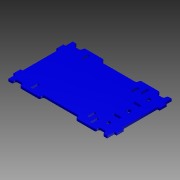
# Autodesk Inventor part: OpenROV 2.3 Dev EChassis Main Plate
Saved by Autodesk Inventor 2012 (Build 160160000, 160)
## iProperties
Created: 2011-12-20
Part Number: OpenROV 2.3 Dev EChassis Main Plate
Document SubType Name: Modeling
Designer: user
Density: 1 g/cm^3
Material: Default
Author: user
Autodesk Inventor part; units mm, degrees
ref_plane "YZ Plane" through (0, 0, 0) normal (1, 0, 0) x (0, 1, 0)
ref_plane "XZ Plane" through (0, 0, 0) normal (0, 1, 0) x (-1, 0, 0)
ref_plane "XY Plane" through (0, 0, 0) normal (0, 0, 1) x (1, 0, 0)
sketch "Sketch1" plane through (0, 0, 0) normal (0, 0, 1) x (1, 0, 0)
  line L0 (138, 80) -> (141, 80)
  line L1 (141, 80) -> (141, 70)
  line L2 (141, 70) -> (138, 70)
  line L3 (138, 10) -> (141, 10)
  line L4 (141, 10) -> (141, 20)
  line L5 (141, 20) -> (138, 20)
  line L6 (138, 80) -> (138, 90)
  line L7 (138, 20) -> (138, 70)
  line L8 (0, 80) -> (-3, 80)
  line L9 (-3, 80) -> (-3, 70)
  line L10 (-3, 70) -> (0, 70)
  line L11 (0, 20) -> (-3, 20)
  line L12 (-3, 20) -> (-3, 10)
  line L13 (-3, 10) -> (0, 10)
  line L14 (0, 90) -> (0, 80)
  line L15 (0, 70) -> (0, 20)
  line L16 (0, 10) -> (0, 0)
  line L17 (26, 85) -> (29, 85)
  line L18 (29, 85) -> (29, 75)
  line L19 (29, 75) -> (26, 75)
  line L20 (26, 75) -> (26, 85)
  line L21 (26, 15) -> (29, 15)
  line L22 (29, 15) -> (29, 5)
  line L23 (29, 5) -> (26, 5)
  line L24 (26, 5) -> (26, 15)
  line L25 (109, 85) -> (112, 85)
  line L26 (112, 85) -> (112, 75)
  line L27 (112, 75) -> (109, 75)
  line L28 (109, 75) -> (109, 85)
  line L29 (109, 15) -> (112, 15)
  line L30 (112, 15) -> (112, 5)
  line L31 (112, 5) -> (109, 5)
  line L32 (109, 5) -> (109, 15)
  line L33 (16, 88) -> (16, 87)
  line L34 (14, 85) -> (8, 85)
  line L35 (6, 87) -> (6, 88)
  line L36 (94, 88) -> (94, 87)
  line L37 (92, 85) -> (46, 85)
  line L38 (44, 87) -> (44, 88)
  line L39 (132, 88) -> (132, 87)
  line L40 (130, 85) -> (124, 85)
  line L41 (122, 87) -> (122, 88)
  line L42 (138, 90) -> (134, 90)
  line L43 (0, 90) -> (4, 90)
  line L44 (18, 90) -> (42, 90)
  line L45 (96, 90) -> (120, 90)
  line L46 (16, 2) -> (16, 3)
  line L47 (14, 5) -> (8, 5)
  line L48 (6, 3) -> (6, 2)
  line L49 (94, 2) -> (94, 3)
  line L50 (92, 5) -> (46, 5)
  line L51 (44, 3) -> (44, 2)
  line L52 (132, 2) -> (132, 3)
  line L53 (130, 5) -> (124, 5)
  line L54 (122, 3) -> (122, 2)
  line L55 (96, 0) -> (120, 0)
  line L56 (0, 0) -> (4, 0)
  line L57 (18, 0) -> (42, 0)
  arc A0 (4, 0) -> (6, 2) centre (4, 2) ccw
  arc A1 (8, 5) -> (6, 3) centre (8, 3) ccw
  arc A2 (16, 3) -> (14, 5) centre (14, 3) ccw
  arc A3 (16, 2) -> (18, 0) centre (18, 2) ccw
  arc A4 (42, 0) -> (44, 2) centre (42, 2) ccw
  arc A5 (46, 5) -> (44, 3) centre (46, 3) ccw
  arc A6 (94, 3) -> (92, 5) centre (92, 3) ccw
  arc A7 (94, 2) -> (96, 0) centre (96, 2) ccw
  arc A8 (120, 0) -> (122, 2) centre (120, 2) ccw
  arc A9 (124, 5) -> (122, 3) centre (124, 3) ccw
  arc A10 (132, 3) -> (130, 5) centre (130, 3) ccw
  arc A11 (132, 2) -> (134, 0) centre (134, 2) ccw
  arc A12 (6, 88) -> (4, 90) centre (4, 88) ccw
  arc A13 (6, 87) -> (8, 85) centre (8, 87) ccw
  arc A14 (14, 85) -> (16, 87) centre (14, 87) ccw
  arc A15 (18, 90) -> (16, 88) centre (18, 88) ccw
  arc A16 (44, 88) -> (42, 90) centre (42, 88) ccw
  arc A17 (44, 87) -> (46, 85) centre (46, 87) ccw
  arc A18 (92, 85) -> (94, 87) centre (92, 87) ccw
  arc A19 (96, 90) -> (94, 88) centre (96, 88) ccw
  arc A20 (122, 88) -> (120, 90) centre (120, 88) ccw
  arc A21 (122, 87) -> (124, 85) centre (124, 87) ccw
  arc A22 (130, 85) -> (132, 87) centre (130, 87) ccw
  arc A23 (134, 90) -> (132, 88) centre (134, 88) ccw
  line L58 (138, 10) -> (138, 0)
  line L59 (138, 0) -> (134, 0)
  line L60 (103, 10) -> (100, 10)
  line L61 (100, 10) -> (100, 20)
  line L62 (100, 20) -> (103, 20)
  line L63 (103, 20) -> (103, 10)
  line L64 (103, 80) -> (100, 80)
  line L65 (100, 80) -> (100, 70)
  line L66 (100, 70) -> (103, 70)
  line L67 (103, 70) -> (103, 80)
  line L68 (115.5, 60.5) -> (125.5, 60.5)
  line L69 (125.5, 60.5) -> (125.5, 57.5)
  line L70 (125.5, 57.5) -> (115.5, 57.5)
  line L71 (115.5, 57.5) -> (115.5, 60.5)
  line L72 (115.5, 32.5) -> (125.5, 32.5)
  line L73 (125.5, 32.5) -> (125.5, 29.5)
  line L74 (125.5, 29.5) -> (115.5, 29.5)
  line L75 (115.5, 29.5) -> (115.5, 32.5)
  circle A24 centre (123, 45) radius 2.5
  circle A25 centre (123, 73) radius 2.5
  circle A26 centre (123, 17) radius 2.5
  point P0 (16, 85)
  point P1 (6, 85)
  point P2 (94, 85)
  point P3 (44, 85)
  point P4 (132, 85)
  point P5 (122, 85)
  point P6 (16, 5)
  point P7 (6, 5)
  point P8 (94, 5)
  point P9 (44, 5)
  point P10 (132, 5)
  point P11 (122, 5)
  dimension "d1" = 90
  dimension "d3" = 10
  dimension "d4" = 50
  dimension "d5" = 10
  dimension "d10" = 3
  dimension "d11" = 3
  dimension "d13" = 3
  dimension "d14" = 3
  dimension "d16" = 10
  dimension "d17" = 10
  dimension "d20" = 138
  dimension "d21" = 50
  dimension "d22" = 3
  dimension "d23" = 3
  dimension "d24" = 3
  dimension "d27" = 26
  dimension "d28" = 3
  dimension "d30" = 3
  dimension "d31" = 26
  dimension "d33" = 10
  dimension "d34" = 10
  dimension "d35" = 26
  dimension "d36" = 3
  dimension "d38" = 10
  dimension "d39" = 3
  dimension "d40" = 10
  dimension "d45" = 10
  dimension "d46" = 50
  dimension "d47" = 10
  dimension "d48" = 6
  dimension "d49" = 6
  dimension "d54" = 10
  dimension "d55" = 50
  dimension "d56" = 10
  dimension "d57" = 2
  dimension "d58" = 26
  dimension "d59" = 6
  dimension "d60" = 6
  dimension "d62" = 28
  dimension "d63" = 3
  dimension "d64" = 28
  dimension "d65" = 28
  dimension "d66" = 28
  dimension "d67" = 5
  dimension "d68" = 5
  dimension "d69" = 5
  dimension "d70" = 5
  dimension "d71" = 5
  dimension "d72" = 5
  dimension "d73" = 5
  dimension "d74" = 5
  dimension "d75" = 5
  dimension "d76" = 5
  dimension "d77" = 5
  dimension "d78" = 5
  dimension "d79" = 3
  dimension "d80" = 10
  dimension "d81" = 35
  dimension "d82" = 10
  dimension "d83" = 3
  dimension "d84" = 10
  dimension "d85" = 10
  dimension "d86" = 35
  dimension "d89" = 10
  constraints: 152 end point, 48 point on circle, 48 tangent, 35 parallel, 27 centre point, 24 point on line, 23 equal radius, 20 perpendicular, 15 horizontal, 3 collinear
  measures "d1" distance of L14.start L16.end
  measures "d3" distance between parallel lines of L2 L0
  measures "d4" distance between parallel lines of L5 L2
  measures "d5" distance between parallel lines of L5 L3
  measures "d10" distance between parallel lines of L7 L4
  measures "d11" distance between parallel lines of L7 L1
  measures "d13" distance of L8.start L8.end
  measures "d14" distance between parallel lines of L16 L12
  measures "d16" distance of L8.end L9.end
  measures "d17" distance of L11.end L12.end
  measures "d20" distance between parallel lines of L15 L7
  measures "d21" distance of L10.end L11.start
  measures "d22" distance of L11.start L11.end
  measures "d23" distance of L3.start L3.end
  measures "d24" distance between parallel lines of L1 L6
  measures "d27" distance between parallel lines of L14 L20
  measures "d28" distance of L17.start L17.end
  measures "d30" distance of L21.start L21.end
  measures "d31" distance between parallel lines of L16 L24
  measures "d33" distance of L17.end L18.end
  measures "d34" distance of L21.end L22.end
  measures "d35" distance between parallel lines of L6 L26
  measures "d36" distance of L25.start L25.end
  measures "d38" distance of L27.end L25.start
  measures "d39" distance of L29.start L29.end
  measures "d40" distance of L31.end L29.start
  measures "d45" distance of point (16, 85) point (6, 85)
  measures "d46" distance of point (94, 85) point (44, 85)
  measures "d47" distance of point (132, 85) point (122, 85)
  measures "d48" distance between parallel lines of L14 L35
  measures "d49" distance between parallel lines of L6 L39
  measures "d54" distance of point (16, 5) point (6, 5)
  measures "d55" distance of point (94, 5) point (44, 5)
  measures "d56" distance of point (132, 5) point (122, 5)
  measures "d57" radius of A0
  measures "d58" distance between parallel lines of L58 L30
  measures "d59" distance between parallel lines of L16 L48
  measures "d60" distance between parallel lines of L58 L52
  measures "d62" distance between parallel lines of L41 L36
  measures "d63" distance of L9.end L10.end
  measures "d64" distance between parallel lines of L38 L33
  measures "d65" distance between parallel lines of L51 L46
  measures "d66" distance between parallel lines of L49 L54
  measures "d67" distance between parallel lines of L56 L47
  measures "d68" distance between parallel lines of L47 L57
  measures "d69" distance between parallel lines of L50 L57
  measures "d70" distance between parallel lines of L55 L50
  measures "d71" distance between parallel lines of L34 L43
  measures "d72" distance between parallel lines of L44 L34
  measures "d73" distance between parallel lines of L37 L44
  measures "d74" distance between parallel lines of L37 L45
  measures "d75" distance between parallel lines of L55 L31
  measures "d76" distance between parallel lines of L25 L45
  measures "d77" distance between parallel lines of L44 L17
  measures "d78" distance between parallel lines of L57 L23
  measures "d79" distance of L61.end L62.end
  measures "d80" distance of L60.end L61.end
  measures "d81" distance between parallel lines of L7 L63
  measures "d82" distance between parallel lines of L55 L60
  measures "d83" distance of L65.end L66.end
  measures "d84" distance of L64.end L65.end
  measures "d85" distance between parallel lines of L45 L64
  measures "d86" distance between parallel lines of L7 L67
  measures "d89" distance of L69.end L70.end
extrude "Extrusion5" add sketch "Sketch1" along normal blind 3
body "Solid5"
